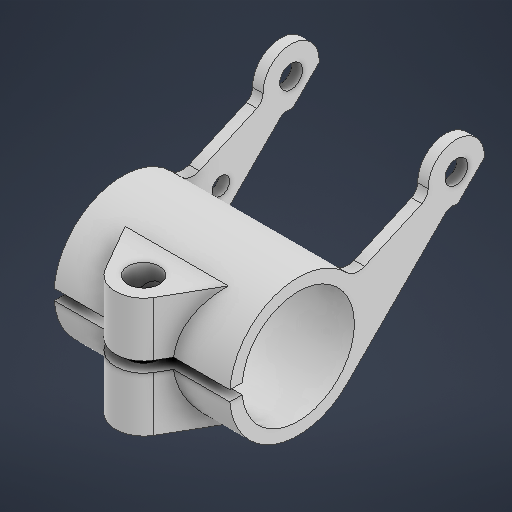
# Autodesk Inventor part: 28
Saved by Autodesk Inventor 2026.2 (Build 302298010, 298A)
## iProperties
Created: 2026-03-18
Part Number: 28
Material: Generico
Document SubType Name: Modeling
Designer: mahsa
Density: 1 g/cm^3
Appearance: Default
Author: mahsa
Autodesk Inventor part; units mm, degrees
note: some values were not read from the file. Chosen so that the rebuilt part matches the saved one: second side of "Estrusione1".
ref_plane "XZ Plane" through (0, 0, 0) normal (0, 1, 0) x (-1, 0, 0)
ref_plane "XY Plane" through (0, 0, 0) normal (0, 0, 1) x (1, 0, 0)
sketch "Schizzo1" plane through (0, 0, 0) normal (1, 0, 0) x (0, 1, 0)
  circle A0 centre (46, -90) radius 6.5
  line L0 (46, -90) -> (62, -90) construction
  line L1 (56.3823, -102.1741) -> (55.8415, -102.7149)
  line L2 (44.998, -105.9686) -> (30.0314, -91.002)
  arc A1 (30.1242, -88.0102) -> (28.6986, -83.8529) centre (25.163, -87.3884) ccw
  line L3 (-27.5772, -27.5772) -> (28.6986, -83.8529)
  line L4 (-5.3717, -38.6283) -> (57.3137, -101.3137) construction
  line L5 (46, -90) -> (62, -90) construction
  line L6 (25.5345, -37.7726) -> (40.0364, -70.4397)
  arc A2 (27.4303, -27.7232) -> (25.5345, -37.7726) centre (33.7604, -34.1209) ccw
  arc A3 (40.0364, -70.4397) -> (45.6511, -74.0038) centre (45.5203, -68.0052) ccw
  arc A4 (44.998, -105.9686) -> (45.6511, -74.0038) centre (46, -90) ccw
  arc A5 (30.1242, -88.0102) -> (30.0314, -91.002) centre (46, -90) ccw
  circle A6 centre (0, 0) radius 39
  dimension "d9" = 46
  dimension "d10" = 90
  dimension "d11" = 13
  dimension "d14" = 10
  dimension "d16" = 45
  dimension "d18" = 18
  dimension "d19" = 12
  dimension "d40" = 78
  constraints: 14 end point, 12 point on circle, 7 centre point, 5 tangent, 2 coincident, 2 horizontal, 1 perpendicular, 1 point on line, 2 other
  measures "d9" horizontal distance of A4.centre point (0, 0)
  measures "d10" vertical distance of A4.centre point (0, 0)
  measures "d11" diameter of A0
  measures "d14" diameter of A1
  measures "d16" angle of L4 L5
  measures "d18" diameter of A2
  measures "d19" diameter of A3
  measures "d40" diameter of A6
extrude "Estrusione1" add sketch "Schizzo1" against normal blind 100 contours A6
extrude "Estrusione2" add sketch "Schizzo1" against normal blind 6 contours L2 A5 A1 L3 A6 A2 L6 A3 A4
ref_plane "Piano di lavoro1" through (-100, 0, 0) normal (1, 0, 0) x (0, 1, 0)
sketch "Schizzo2" plane through (-100, 0, 0) normal (1, 0, 0) x (0, 1, 0)
  arc A0 (44.998, -105.9686) -> (45.6511, -74.0038) centre (46, -90) ccw projected
  circle A1 centre (46, -90) radius 6.5 projected
  line L0 (44.998, -105.9686) -> (30.0314, -91.002) projected
  line L1 (25.5345, -37.7726) -> (40.0364, -70.4397) projected
  arc A2 (40.0364, -70.4397) -> (45.6511, -74.0038) centre (45.5203, -68.0052) ccw projected
  line L2 (28.6986, -83.8529) -> (-27.5772, -27.5772) projected
  arc A3 (30.1242, -88.0102) -> (28.6986, -83.8529) centre (25.163, -87.3884) ccw projected
  arc A4 (30.1242, -88.0102) -> (30.0314, -91.002) centre (46, -90) ccw projected
  arc A5 (27.4303, -27.7232) -> (25.5345, -37.7726) centre (33.7604, -34.1209) ccw projected
  arc A6 (-27.5772, -27.5772) -> (27.4303, -27.7232) centre (0, 0) ccw projected
  line L3 (0, 0) -> (0, -50)
  line L4 (0, -50) -> (12, -50)
  circle A7 centre (12, -50) radius 5
  dimension "d27" = 50
  dimension "d28" = 12
  dimension "d29" = 10
  constraints: 4 end point, 1 centre point, 1 coincident, 1 perpendicular, 1 vertical
  measures "d27" distance of L3.start L3.end
  measures "d28" distance of L3.end L4.end
  measures "d29" diameter of A7
extrude "Estrusione3" add sketch "Schizzo2" along normal blind 6
sketch "Schizzo4" plane through (0, 0, 0) normal (0, 1, 0) x (-1, 0, 0)
  line L0 (0, 39) -> (100, 39) projected
  line L1 (9.5855, 0) -> (50, 0)
  line L2 (50, 0) -> (50, 38)
  circle A0 centre (50, 38) radius 9
  arc A1 (63.8564, 46) -> (36.1436, 46) centre (50, 38) ccw
  line L3 (50, 0) -> (90.4145, 0)
  line L4 (90.4145, 0) -> (63.8564, 46)
  line L5 (9.5855, 0) -> (36.1436, 46)
  line L6 (50, 38) -> (50, 54) construction
  point P0 (0, 0)
  point P1 (65.9687, 39)
  point P2 (34.0313, 39)
  point P3 (41.0557, 39)
  point P4 (58.9443, 39)
  point P5 (32.1021, 39)
  point P6 (67.8979, 39)
  dimension "d42" = 50
  dimension "d43" = 38
  dimension "d44" = 18
  dimension "d45" = 32
  dimension "d49" = 60
  constraints: 12 end point, 3 point on circle, 2 centre point, 2 coincident, 2 horizontal, 2 tangent, 1 perpendicular, 1 vertical
  measures "d42" distance of point (0, 0) L1.end
  measures "d43" distance of L1.end L2.end
  measures "d44" diameter of A0
  measures "d45" diameter of A1
  measures "d49" angle of L5 L4
extrude "Estrusione4" add sketch "Schizzo4" along normal mid plane 68 contours L5 A1 L4 L0 A0 | L0 A0 L2 L1 L5 | L0 L4 L3 L2 A0
sketch "Schizzo6" plane through (0, 0, 0) normal (1, 0, 0) x (0, 1, 0)
  line L0 (-3, 31.8591) -> (-3, 54)
  line L1 (-34, 54) -> (34, 54) projected
  line L2 (-3, 54) -> (3, 54)
  line L3 (3, 54) -> (3, 31.8591)
  circle A0 centre (0, 0) radius 32
  circle A1 centre (0, 0) radius 39
  dimension "d55" = 6
  dimension "d56" = 64
  dimension "d57" = 78
  constraints: 6 end point, 2 centre point, 2 coincident, 2 point on circle, 2 point on line, 1 perpendicular
  measures "d55" distance of L0.end L2.end
  measures "d56" diameter of A0
  measures "d57" diameter of A1
extrude "Estrusione5" cut sketch "Schizzo6" against normal up to next contours L0 A1 L3 A0 | A0 | L0 L1 L3 A1 picked at (2.3338, 34.2426)
